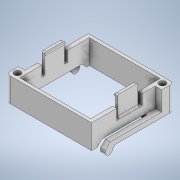
# Autodesk Inventor part: cuadrado
Saved by Autodesk Inventor 2020 (Build 240168000, 168)
## iProperties
Created: 2020-08-05
Part Number: cuadrado
Material: Generic
Document SubType Name: Modeling
Designer: Samuel
Density: 1 g/cm^3
Appearance: Default
Author: Samuel
Autodesk Inventor part; units mm, degrees
ref_plane "YZ Plane" through (0, 0, 0) normal (1, 0, 0) x (0, 1, 0)
ref_plane "XZ Plane" through (0, 0, 0) normal (0, 1, 0) x (-1, 0, 0)
ref_plane "XY Plane" through (0, 0, 0) normal (0, 0, 1) x (1, 0, 0)
sketch "Sketch1" plane through (0, 0, 0) normal (0, 1, 0) x (-1, 0, 0)
  line L0 (-24.5, 23.5) -> (24.5, 23.5)
  line L1 (24.5, 23.5) -> (24.5, -23.5)
  line L2 (24.5, -23.5) -> (-24.5, -23.5)
  line L3 (-24.5, -23.5) -> (-24.5, 23.5)
  line L4 (-24.5, 23.5) -> (24.5, -23.5) construction
  line L5 (24.5, 23.5) -> (-24.5, -23.5) construction
  line L6 (24.5, 23.5) -> (22, 23.5)
  line L7 (22, 23.5) -> (22, -23.5)
  line L8 (22, -23.5) -> (24.5, -23.5)
  line L9 (24.5, -23.5) -> (24.5, 23.5)
  line L10 (24.5, -23.5) -> (-24.5, -23.5)
  line L11 (-24.5, -23.5) -> (-24.5, -21.6)
  line L12 (-24.5, -21.6) -> (24.5, -21.6)
  line L13 (24.5, -21.6) -> (24.5, -23.5)
  line L14 (-24.5, -23.5) -> (-22, -23.5)
  line L15 (-22, -23.5) -> (-22, 23.5)
  line L16 (-22, 23.5) -> (-24.5, 23.5)
  line L17 (-24.5, 23.5) -> (-24.5, -23.5)
  line L18 (-24.5, 23.5) -> (24.5, 23.5)
  line L19 (24.5, 23.5) -> (24.5, 21.6)
  line L20 (24.5, 21.6) -> (-24.5, 21.6)
  line L21 (-24.5, 21.6) -> (-24.5, 23.5)
  point P0 (0, 0)
  point P1 (-22, -21.6)
  point P2 (-22, 21.6)
  point P3 (22, 21.6)
  point P4 (22, -21.6)
  dimension "d0" = 49
  dimension "d1" = 47
  dimension "d2" = 2.5
  dimension "d3" = 1.9
  dimension "d4" = 2.5
  dimension "d5" = 1.9
  constraints: 44 end point, 10 parallel, 5 horizontal, 5 perpendicular, 4 point on line, 2 midpoint
  measures "d0" distance of L1.end L2.end
  measures "d1" distance of L0.end L1.end
  measures "d2" distance of L8.end L7.end
  measures "d3" distance of L10.end L11.end
  measures "d4" distance of L16.end L15.end
  measures "d5" distance of L18.end L19.end
extrude "Extrusion1" add sketch "Sketch1" along normal blind 15 contours L0 L15 L20 L3 | L0 L7 L20 L15 | L20 L15 L12 L3 | L0 L1 L20 L7 | L12 L15 L2 L3 | L20 L1 L12 L7 | L12 L7 L2 L15 | L12 L1 L2 L7
sketch "Sketch2" plane through (0, 15, 0) normal (0, 1, 0) x (1, 0, 0)
  line L0 (24.5, 23.5) -> (-24.5, 23.5) projected
  line L1 (22, 23.5) -> (28.5, 23.5)
  line L2 (28.5, 23.5) -> (28.5, 16)
  line L3 (28.5, 16) -> (22, 16)
  line L4 (22, 16) -> (22, 23.5)
  line L5 (22, 23.5) -> (28.5, 23.5)
  line L6 (28.5, 23.5) -> (28.5, 16)
  line L7 (-24.5, -23.5) -> (24.5, -23.5) projected
  line L8 (-22, -23.5) -> (-28.5, -23.5)
  line L9 (-28.5, -23.5) -> (-28.5, -16)
  line L10 (-28.5, -16) -> (-22, -16)
  line L11 (-22, -16) -> (-22, -23.5)
  point P0 (0, 0)
  dimension "d8" = 6.5
  dimension "d9" = 6.5
  constraints: 20 end point, 4 parallel, 3 perpendicular, 2 horizontal, 2 point on line, 1 collinear
  measures "d8" distance of L1.start L1.end
  measures "d9" distance of L9.end L10.end
extrude "Extrusion2" add sketch "Sketch2" against normal blind 15
sketch "Sketch3" plane through (0, 15, 0) normal (0, 1, 0) x (1, 0, 0)
  line L0 (-28.5, -23.5) -> (24.5, -23.5) projected
  line L1 (24.5, -23.5) -> (24.5, 16) projected
  line L2 (24.5, 16) -> (28.5, 16) projected
  line L3 (28.5, 16) -> (28.5, 23.5) projected
  line L4 (28.5, 23.5) -> (-24.5, 23.5) projected
  line L5 (-24.5, 23.5) -> (-24.5, -16) projected
  line L6 (-24.5, -16) -> (-28.5, -16) projected
  line L7 (-28.5, -16) -> (-28.5, -23.5) projected
  line L8 (-22, -21.6) -> (-22, 21.6) projected
  line L9 (-22, 21.6) -> (22, 21.6) projected
  line L10 (22, 21.6) -> (22, -21.6) projected
  line L11 (22, -21.6) -> (-22, -21.6) projected
  line L12 (28.5, 23.5) -> (28.5, 16) projected
  line L13 (22, 23.5) -> (28.5, 23.5)
  line L14 (28.5, 23.5) -> (28.5, 16)
  line L15 (28.5, 16) -> (22, 16)
  line L16 (22, 16) -> (22, 23.5)
  line L17 (-28.5, -16) -> (-24.5, -16) projected
  line L18 (-28.5, -23.5) -> (24.5, -23.5) projected
  line L19 (-28.5, -16) -> (-22, -16)
  line L20 (-22, -16) -> (-22, -23.5)
  line L21 (-22, -23.5) -> (-28.5, -23.5)
  line L22 (-28.5, -23.5) -> (-28.5, -16)
  circle A0 centre (25.25, 19.75) radius 1
  circle A1 centre (-25.25, -19.75) radius 1
  point P0 (0, 0)
  dimension "d12" = 2
  dimension "d13" = 2
  constraints: 16 end point, 4 parallel, 2 centre point, 2 coincident, 2 horizontal, 2 perpendicular, 2 point on line
  measures "d12" diameter of A0
  measures "d13" diameter of A1
extrude "Extrusion3" cut sketch "Sketch3" against normal blind 15 contours A0 | A1
sketch "Sketch4" plane through (0, 15, 0) normal (0, 1, 0) x (1, 0, 0)
  circle A0 centre (25.25, 19.75) radius 1 projected
  circle A1 centre (-25.25, -19.75) radius 1 projected
  circle A2 centre (-25.25, -19.75) radius 2
  circle A3 centre (25.25, 19.75) radius 2
  point P0 (0, 0)
  dimension "d16" = 4
  dimension "d17" = 4
  constraints: 2 centre point, 2 coincident
  measures "d16" diameter of A2
  measures "d17" diameter of A3
extrude "Extrusion4" cut sketch "Sketch4" against normal blind 4
sketch "Sketch5" plane through (0, 0, 0) normal (0, -1, 0) x (1, 0, 0)
  circle A0 centre (25.25, -19.75) radius 2 projected
  circle A1 centre (-25.25, 19.75) radius 2 projected
  point P0 (0, 0)
extrude "Extrusion5" cut sketch "Sketch5" against normal blind 4
fillet "Fillet1" radius 2.5 2 edges at (28.5, 7.5, -23.5) (-28.5, 7.5, 23.5)
sketch "Sketch6" plane through (0, 15, 0) normal (0, 1, 0) x (1, 0, 0)
  arc A0 (-28.5, -21) -> (-26, -23.5) centre (-26, -21) ccw projected
  line L0 (-26, -23.5) -> (24.5, -23.5) projected
  line L1 (24.5, -23.5) -> (24.5, 16) projected
  line L2 (24.5, 16) -> (28.5, 16) projected
  line L3 (28.5, 16) -> (28.5, 21) projected
  arc A1 (28.5, 21) -> (26, 23.5) centre (26, 21) ccw projected
  line L4 (26, 23.5) -> (-24.5, 23.5) projected
  line L5 (-24.5, 23.5) -> (-24.5, -16) projected
  line L6 (-24.5, -16) -> (-28.5, -16) projected
  line L7 (-28.5, -16) -> (-28.5, -21) projected
  circle A2 centre (-25.25, -19.75) radius 2 projected
  circle A3 centre (25.25, 19.75) radius 2 projected
  line L8 (-22, -21.6) -> (-22, 21.6) projected
  line L9 (-22, 21.6) -> (22, 21.6) projected
  line L10 (22, 21.6) -> (22, -21.6) projected
  line L11 (22, -21.6) -> (-22, -21.6) projected
  line L12 (26, 23.5) -> (-24.5, 23.5) projected
  line L13 (24.5, -23.5) -> (24.5, 16) projected
  line L14 (22, 23.5) -> (24.5, 23.5)
  line L15 (24.5, 23.5) -> (24.5, -23.5)
  line L16 (24.5, -23.5) -> (22, -23.5)
  line L17 (22, -23.5) -> (22, 23.5)
  line L18 (-22, -23.5) -> (-24.5, -23.5)
  line L19 (-24.5, -23.5) -> (-24.5, 23.5)
  line L20 (-24.5, 23.5) -> (-22, 23.5)
  line L21 (-22, 23.5) -> (-22, -23.5)
  line L22 (-22, -21.6) -> (-22, 21.6) projected
  line L23 (-24.5, -8) -> (-22, -8)
  line L24 (-22, -8) -> (-22, 8)
  line L25 (-22, 8) -> (-24.5, 8)
  line L26 (-24.5, 8) -> (-24.5, -8)
  line L27 (-24.5, -8) -> (-22, 8) construction
  line L28 (-22, -8) -> (-24.5, 8) construction
  line L29 (22, -8) -> (24.5, -8)
  line L30 (24.5, -8) -> (24.5, 8)
  line L31 (24.5, 8) -> (22, 8)
  line L32 (22, 8) -> (22, -8)
  line L33 (22, -8) -> (24.5, 8) construction
  line L34 (24.5, -8) -> (22, 8) construction
  point P0 (0, 0)
  point P1 (-23.25, 0)
  point P2 (23.25, 0)
  dimension "d23" = 16
  dimension "d24" = 16
  constraints: 40 end point, 8 parallel, 4 horizontal, 4 midpoint, 4 perpendicular, 4 point on line
  measures "d23" distance of L24.end L23.end
  measures "d24" distance of L30.end L29.end
extrude "Extrusion6" cut sketch "Sketch6" against normal blind 6.5 contours L5 L25 L8 L23 | L29 L10 L31 L1
sketch "Sketch7" plane through (0, 8.5, 0) normal (0, 1, 0) x (1, 0, 0)
  line L0 (-22, -21.6) -> (-22, 21.6) projected
  line L1 (-22, 0) -> (-22, 6.25)
  line L2 (-22, 6.25) -> (-23.5, 6.25)
  line L3 (-23.5, 6.25) -> (-23.5, -6.25)
  line L4 (-23.5, -6.25) -> (-22, -6.25)
  line L5 (-22, -6.25) -> (-22, 6.25)
  line L6 (22, 21.6) -> (22, -21.6) projected
  line L7 (22, 6.25) -> (23.5, 6.25)
  line L8 (23.5, 6.25) -> (23.5, -6.25)
  line L9 (23.5, -6.25) -> (22, -6.25)
  line L10 (22, -6.25) -> (22, 6.25)
  point P0 (0, 0)
  dimension "d27" = 6.25
  dimension "d28" = 1.5
  dimension "d29" = 12.5
  dimension "d30" = 1.5
  dimension "d31" = 12.5
  constraints: 18 end point, 4 parallel, 2 horizontal, 2 perpendicular, 2 point on line, 1 midpoint
  measures "d27" distance of L1.start L1.end
  measures "d28" distance of L4.end L3.end
  measures "d29" distance of L3.end L2.end
  measures "d30" distance of L8.end L9.end
  measures "d31" distance of L7.end L8.end
extrude "Extrusion7" add sketch "Sketch7" along normal blind 12.5
sketch "Sketch8" plane through (22, 8.5, 6.25) normal (0, 0, 1) x (1, 0, 0)
  line L0 (0, 0) -> (0, 12.5) projected
  line L1 (0, 12.5) -> (0, 11.5)
  line L2 (0, 11.5) -> (-1, 11.5)
  line L3 (0, 11.5) -> (0, 10.5)
  line L4 (0, 10.5) -> (-1, 11.5)
  line L5 (-44, 0) -> (-44, 12.5) projected
  line L6 (-44, 12.5) -> (-44, 11.5)
  line L7 (-44, 11.5) -> (-43, 11.5)
  line L8 (-43, 11.5) -> (-44, 10.5)
  line L9 (-44, 10.5) -> (-44, 11.5)
  point P0 (-22, -8.5)
  dimension "d34" = 1
  dimension "d35" = 1
  dimension "d36" = 1
  dimension "d37" = 1
  dimension "d38" = 1
  constraints: 16 end point, 4 point on line, 3 perpendicular, 1 collinear
  measures "d34" distance of L0.end L1.end
  measures "d35" distance of L1.end L2.end
  measures "d36" distance of L1.end L3.end
  measures "d37" distance of L5.end L6.end
  measures "d38" distance of L6.end L7.end
extrude "Extrusion8" add sketch "Sketch8" against normal blind 12.5
fillet "Fillet2" radius 1 6 edges at (-22.75, 21, 6.25) (-22.75, 21, -6.25) (22.75, 21, 6.25) (22.75, 21, -6.25) (23.5, 8.5, 0) (-23.5, 8.5, 0)
sketch "Sketch9" plane through (24.5, 15, -16) normal (0, 0, 1) x (1, 0, 0)
  line L0 (4, -15) -> (0, -15)
  line L1 (0, -15) -> (0, -12)
  line L2 (0, -12) -> (4, -12)
  line L3 (4, -12) -> (4, -15)
  point P0 (-24.5, -15)
  dimension "d42" = 3
  constraints: 8 end point, 2 parallel, 1 horizontal, 1 perpendicular
  measures "d42" distance of L0.end L1.end
extrude "Extrusion9" add sketch "Sketch9" along normal blind 6
sketch "Sketch11" plane through (-24.5, 15, 16) normal (0, 0, -1) x (-1, 0, 0)
  line L0 (4, -15) -> (0, -15) projected
  line L1 (0, -15) -> (4, -15)
  line L2 (4, -15) -> (4, -12)
  line L3 (4, -12) -> (0, -12)
  line L4 (0, -12) -> (0, -15)
  point P0 (-24.5, -15)
  constraints: 8 end point, 2 parallel, 1 horizontal, 1 perpendicular
extrude "Extrusion10" add sketch "Sketch11" along normal blind 6
sketch "Sketch12" plane through (-24.5, 15, 10) normal (0, 0, -1) x (-1, 0, 0)
  line L0 (0, -12) -> (4, -12) projected
  line L1 (4, -15) -> (1, -15)
  line L2 (1, -15) -> (1, -12)
  line L3 (1, -12) -> (4, -12)
  line L4 (4, -12) -> (4, -15)
  point P0 (-24.5, -15)
  dimension "d47" = 3
  constraints: 8 end point, 2 parallel, 1 horizontal, 1 perpendicular, 1 point on line
  measures "d47" distance of L2.end L3.end
extrude "Extrusion11" add sketch "Sketch12" along normal blind 29
chamfer "Chamfer1" distance 3 angle 45 1 edges at (-27, 3, -19)
sketch "Sketch13" plane through (-28.5, 15, 16) normal (-1, 0, 0) x (0, 0, 1)
  line L0 (-35, -15) -> (-32, -12) projected
  line L1 (-35, -15) -> (-29, -15)
  line L2 (-37, -15) -> (-26, -15) projected
  line L3 (-29, -15) -> (-30.4142, -16.4142)
  line L4 (-30.4142, -16.4142) -> (-35, -16.4142)
  line L5 (-35, -16.4142) -> (-35, -15)
  arc A0 (-35, -16.4142) -> (-30.4142, -16.4142) centre (-32.7071, -16.4142) ccw
  point P0 (-16, -15)
  dimension "d53" = 6
  dimension "d54" = 2
  dimension "d55" = 45
  constraints: 8 end point, 2 point on circle, 1 centre point, 1 parallel, 1 perpendicular, 1 point on line, 1 tangent
  measures "d53" distance of L0.start L1.end
  measures "d54" distance of L1.end L3.end
  measures "d55" angle of L1 L3
extrude "Extrusion12" add sketch "Sketch13" against normal blind 3
sketch "Sketch14" plane through (24.5, 15, -10) normal (0, 0, 1) x (1, 0, 0)
  line L0 (4, -15) -> (4, -12) projected
  line L1 (4, -12) -> (0, -12) projected
  line L2 (0, -15) -> (0, -12) projected
  line L3 (0, -15) -> (4, -15) projected
  line L4 (4, -12) -> (0, -12) projected
  line L5 (4, -15) -> (1, -15)
  line L6 (1, -15) -> (1, -12)
  line L7 (1, -12) -> (4, -12)
  line L8 (4, -12) -> (4, -15)
  point P0 (1, -12)
  point P1 (1, -15)
  constraints: 8 end point, 2 parallel, 1 horizontal, 1 perpendicular, 1 point on line
extrude "Extrusion13" add sketch "Sketch14" along normal blind 29 contours L3 L6 L1 L0
chamfer "Chamfer2" distance 3 angle 45 1 edges at (27, 3, 19)
sketch "Sketch15" plane through (28.5, 15, -16) normal (1, 0, 0) x (0, 0, -1)
  line L0 (-35, -15) -> (-32, -12) projected
  line L1 (5, -15) -> (-35, -15) projected
  line L2 (5, 0) -> (5, -15) projected
  line L3 (0, 0) -> (5, 0) projected
  line L4 (0, 0) -> (0, -12) projected
  line L5 (0, -12) -> (-32, -12) projected
  line L6 (-32, -12) -> (-35, -15) projected
  line L7 (-35, -15) -> (-29, -15)
  line L8 (5.6, -15) -> (-37.6, -15) projected
  line L9 (-29, -15) -> (-30.4142, -16.4142)
  line L10 (-29, -15) -> (-27, -15) construction
  line L11 (-30.4142, -16.4142) -> (-35, -16.4142)
  line L12 (-35, -16.4142) -> (-35, -15)
  arc A0 (-35, -16.4142) -> (-30.4142, -16.4142) centre (-32.7071, -16.4142) ccw
  point P0 (-16, -15)
  dimension "d63" = 6
  dimension "d64" = 2
  dimension "d65" = 135
  constraints: 10 end point, 2 horizontal, 2 point on circle, 1 centre point, 1 equal length, 1 perpendicular, 1 point on line, 1 tangent
  measures "d63" distance of L0.start L7.end
  measures "d64" distance of L7.end L9.end
  measures "d65" angle of L9 L10
extrude "Extrusion14" add sketch "Sketch15" against normal blind 3 contours L1 L9 L11 L12 | L11 A0
sketch "Sketch16" plane through (24.5, 0, 23.5) normal (1, 0, 0) x (0, 0, -1)
  line L0 (33.5, 0) -> (6.5, 0)
  line L1 (6.5, 0) -> (6.5, 3)
  line L2 (6.5, 3) -> (33.5, 3)
  line L3 (33.5, 3) -> (33.5, 0)
  line L4 (6.5, 3) -> (3.4995, 0)
  line L5 (3.4995, 0) -> (6.5, 0)
  line L6 (5.75, 0) -> (5.75, 4) projected
  point P0 (23.5, 0)
  dimension "d68" = 27
  dimension "d69" = 4.243
  constraints: 12 end point, 2 parallel, 2 perpendicular, 1 horizontal
  measures "d68" distance of L1.end L2.end
  measures "d69" distance of L1.end L4.end
extrude "Extrusion15" cut sketch "Sketch16" against normal blind 5
sketch "Sketch17" plane through (-24.5, 0, -23.5) normal (-1, 0, 0) x (0, 0, 1)
  line L0 (33.5, 0) -> (33.5, 3) projected
  line L1 (2.5, 0) -> (36.5, 0) projected
  line L2 (33.5, 3) -> (6.5, 3)
  line L3 (6.5, 3) -> (6.5, 0)
  line L4 (6.5, 0) -> (33.5, 0)
  line L5 (33.5, 0) -> (33.5, 3)
  line L6 (6.5, 3) -> (3.4995, 0)
  line L7 (3.4995, 0) -> (6.5, 0)
  point P0 (23.5, 0)
  dimension "d72" = 27
  dimension "d73" = 4.243
  constraints: 12 end point, 3 point on line, 2 parallel, 1 horizontal, 1 perpendicular
  measures "d72" distance of L4.end L3.end
  measures "d73" distance of L2.end L6.end
extrude "Extrusion16" cut sketch "Sketch17" against normal blind 5
body "Solid1"
